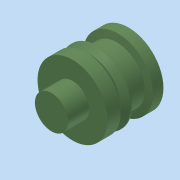
# Autodesk Inventor part: FOX-ME-126-07
Saved by Autodesk Inventor 2014 (Build 180170000, 170)
## iProperties
Created: 2012-08-14
Part Number: FOX-ME-126-07
Document SubType Name: Modeling
Designer: Robert Davis
Density: 2.04 g/cm^3
Material: G10
Mass: 0.153429 g
Surface Area: 1.20744 cm^2
Volume: 0.0752103 cm^3
Description: ANTENNA POST, G10/FR4
Appearance: Olive Green
Author: Robert Davis
Autodesk Inventor part; units mm, degrees
ref_plane "YZ Plane" through (0, 0, 0) normal (1, 0, 0) x (0, 1, 0)
ref_plane "XZ Plane" through (0, 0, 0) normal (0, 1, 0) x (-1, 0, 0)
ref_plane "XY Plane" through (0, 0, 0) normal (0, 0, 1) x (1, 0, 0)
sketch "Sketch1" plane through (0, 0, 0) normal (0, 0, 1) x (1, 0, 0)
  line L0 (0, 0) -> (0, 17.163)
  line L1 (2.5, 4) -> (2.5, 3.25)
  line L2 (2.5, 0) -> (0, 0)
  line L3 (2.5, 3.25) -> (2, 3.1618)
  line L4 (2, 3.1618) -> (2, 1.8382)
  line L5 (2, 1.8382) -> (2.5, 1.75)
  line L6 (0, 0) -> (0, 4)
  line L7 (0, 4) -> (2.5, 4)
  line L8 (2.5, 1.65) -> (2.15, 1.3)
  line L9 (2.15, 1.3) -> (2.5, 0.95)
  line L10 (2.5, 1.75) -> (2.5, 1.65)
  line L11 (2.5, 0.95) -> (2.5, 0)
  dimension "d2" = 5
  dimension "d17" = 0.75
  dimension "d18" = 1.75
  dimension "d19" = 100
  dimension "d20" = 100
  dimension "d24" = 1.3237
  dimension "d39" = 135
  dimension "d40" = 135
  dimension "d41" = 0.35
  dimension "d42" = 1.3
  constraints: 24 end point, 5 vertical, 2 collinear, 2 horizontal, 1 coincident
  measures "d2" diameter of L1 L0
  measures "d17" distance of L1.start L1.end
  measures "d18" distance of L5.end L2.start
  measures "d19" angle of L3 L4
  measures "d20" angle of L4 L5
  measures "d24" distance of L3.end L4.end
  measures "d39" angle of L10 L8
  measures "d40" angle of L11 L9
  measures "d41" distance from line of L11 L8.end
  measures "d42" distance from line of L2 L8.end
revolve "Revolution1" add sketch "Sketch1" angle 360 about axis through (0, 0, 0) along (0, 1, 0)
hole "Hole1" [suppressed]
sketch "Sketch2" plane through (0, 0, 0) normal (0, -1, 0) x (1, 0, 0)
  circle A0 centre (0, 0) radius 1.19
  dimension "d36" = 2.38
  constraints: 1 centre point
  measures "d36" diameter of A0
extrude "Extrusion1" add sketch "Sketch2" along normal blind 1.5
body "Solid1"
